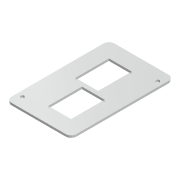
# Autodesk Inventor part: 17-0028-0112
Saved by Autodesk Inventor 2016 SP2 (Build 200236200, 236)
## iProperties
Category: IOP
Company: Universiteit van Amsterdam
Created: 2018-01-26
Part Number: 17-0028-0112
Material: Plastic (perspex PMMA)
Document SubType Name: Modeling
Designer: Daan Giesen
Density: 1.19 g/cm^3
Appearance: Clear
Mass: 10.3779 g
Surface Area: 97.7995 cm^2
Volume: 8.72091 cm^3
Project: Digital PID Loop
Cost Center: 17-0028
User Status: Work in Progress
Authority: Reichsöllner, Lukas
Author: Daan Giesen
Title: Digital PID Loop
Revision Number: A
Autodesk Inventor part; units mm, degrees
ref_plane "YZ Plane" through (0, 0, 0) normal (1, 0, 0) x (0, 1, 0)
ref_plane "XZ Plane" through (0, 0, 0) normal (0, 1, 0) x (-1, 0, 0)
ref_plane "XY Plane" through (0, 0, 0) normal (0, 0, 1) x (1, 0, 0)
sketch "Sketch1" plane through (0, 0, 0) normal (0, 0, 1) x (1, 0, 0)
  line L0 (0, 66.5) -> (0, -66.5) construction
  line L1 (-42, 0) -> (42, 0) construction
  line L2 (30, -47.5) -> (-30, -47.5)
  line L3 (-30, -47.5) -> (-30, 47.5)
  line L4 (-30, 47.5) -> (30, 47.5)
  line L5 (30, 47.5) -> (30, -47.5)
  line L6 (30, -47.5) -> (-30, 47.5) construction
  line L7 (-30, -47.5) -> (30, 47.5) construction
  line L8 (5.5, 2) -> (-15.5, 2)
  line L9 (-15.5, 2) -> (-15.5, 33)
  line L10 (-15.5, 33) -> (5.5, 33)
  line L11 (5.5, 33) -> (5.5, 2)
  line L12 (5.5, 2) -> (-15.5, 33) construction
  line L13 (-15.5, 2) -> (5.5, 33) construction
  line L14 (15.5, -33) -> (-5.5, -33)
  line L15 (-5.5, -33) -> (-5.5, -2)
  line L16 (-5.5, -2) -> (15.5, -2)
  line L17 (15.5, -2) -> (15.5, -33)
  line L18 (15.5, -33) -> (-5.5, -2) construction
  line L19 (-5.5, -33) -> (15.5, -2) construction
  point P0 (0, 0)
  point P1 (-5, 17.5)
  point P2 (5, -17.5)
  dimension "d13" = 95
  dimension "d14" = 60
  dimension "d15" = 31
  dimension "d16" = 21
  dimension "d17" = 5
  dimension "d18" = 17.5
  dimension "d19" = 17.5
  dimension "d20" = 5
  constraints: 36 end point, 8 parallel, 6 midpoint, 3 horizontal, 3 perpendicular
  measures "d13" distance of L4.end L2.start
  measures "d14" distance of L3.end L4.end
  measures "d15" distance of L10.end L8.start
  measures "d16" distance of L9.end L10.end
  measures "d17" horizontal distance of point (0, 0) point (-5, 17.5)
  measures "d18" vertical distance of point (0, 0) point (-5, 17.5)
  measures "d19" vertical distance of point (0, 0) point (5, -17.5)
  measures "d20" horizontal distance of point (0, 0) point (5, -17.5)
extrude "Extrusion3" add sketch "Sketch1" along normal blind 2
sketch "Sketch2" plane through (0, 0, 2) normal (0, 0, 1) x (1, 0, 0)
  line L0 (25, -37.5) -> (-25, -37.5) construction
  line L1 (-25, -37.5) -> (-25, 37.5) construction
  line L2 (-25, 37.5) -> (25, 37.5) construction
  line L3 (25, 37.5) -> (25, -37.5) construction
  line L4 (25, -37.5) -> (-25, 37.5) construction
  line L5 (-25, -37.5) -> (25, 37.5) construction
  point P0 (0, 0)
  point P1 (-25, -37.5)
  dimension "d21" = 75
  dimension "d22" = 50
  constraints: 12 end point, 2 midpoint, 2 parallel, 1 coincident, 1 horizontal, 1 perpendicular, 1 point on line
  measures "d21" distance of L2.end L0.start
  measures "d22" distance of L1.end L2.end
hole "Hole1" at (25, 37.5, 2) at (-25, -37.5, 2) direction (0, 0, -1) diameter 3.2 end through all
fillet "Fillet1" radius 5 4 edges at (30, 47.5, 1) (-30, 47.5, 1) (30, -47.5, 1) (-30, -47.5, 1)
equation "\"d19\" = d18"
equation "\"d20\" = d17"
body "Solid3"
